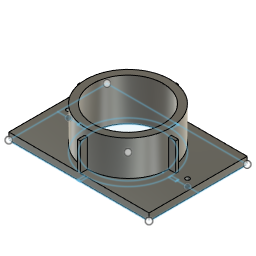
Soporte v1 (Autodesk Fusion 360 design; units mm, degrees)
Autodesk Fusion 360 part; units mm, degrees
sketch "Boceto1" plane through (0, 0, 0) normal (0, 0, 1) x (1, 0, 0)
  circle A0 centre (14.4542, 45.9008) radius 25
  circle A1 centre (14.4542, 45.9008) radius 30
  line L0 (14.4542, 10.9008) -> (15.4542, 10.9008)
  line L1 (15.4542, 10.9008) -> (15.4542, 15.9174)
  line L2 (14.4542, 10.9008) -> (13.4542, 10.9008)
  line L3 (-35.5458, 10.9008) -> (-35.5458, 80.9008)
  line L4 (14.4542, 80.9008) -> (15.4542, 80.9008)
  line L5 (15.4542, 80.9008) -> (15.4542, 75.8841)
  line L6 (15.4542, 80.9008) -> (13.4542, 80.9008)
  line L7 (13.4542, 80.9008) -> (13.4542, 75.8841)
  line L8 (64.4542, 10.9008) -> (64.4542, 80.9008)
  line L9 (14.4542, 10.9008) -> (-35.5458, 10.9008)
  line L10 (14.4542, 10.9008) -> (64.4542, 10.9008)
  line L11 (14.4542, 80.9008) -> (-35.5458, 80.9008)
  line L12 (14.4542, 80.9008) -> (64.4542, 80.9008)
  line L13 (-20.5458, 45.9008) -> (-20.5458, 46.9008)
  line L14 (-20.5458, 46.9008) -> (-15.5291, 46.9008)
  line L15 (-20.5458, 45.9008) -> (-20.5458, 44.9008)
  line L16 (-20.5458, 44.9008) -> (-15.5291, 44.9008)
  line L17 (-20.5458, 45.9008) -> (-35.5458, 45.9008)
  circle A2 centre (-28.0458, 45.9008) radius 1.5
  line L18 (49.4542, 45.9008) -> (49.4542, 46.9008)
  line L19 (49.4542, 46.9008) -> (44.4375, 46.9008)
  line L20 (49.4542, 45.9008) -> (49.4542, 44.9008)
  line L21 (49.4542, 44.9008) -> (44.4375, 44.9008)
  line L22 (49.4542, 45.9008) -> (64.4542, 45.9008)
  circle A3 centre (56.9542, 45.9008) radius 1.5
  line L23 (13.4542, 10.9008) -> (13.4542, 15.9174)
  dimension "d1" = 50
  dimension "d2" = 60
  dimension "d7" = 70
  dimension "d8" = 1
  dimension "d9" = 2
  dimension "d21" = 70
  dimension "d30" = 50
  dimension "d31" = 50
  dimension "d32" = 50
  dimension "d33" = 50
  dimension "d39" = 3
  dimension "d40" = 5.0167
  dimension "d44" = 5.0167
  dimension "d45" = 3
  constraint concentric A0 A1
  constraint coincident A1 L1.end
  constraint perpendicular L0 L1
  constraint coincident A1 L5.end
  constraint perpendicular L4 L5
  constraint coincident A1 L7.end
  constraint parallel L2 L9
  constraint perpendicular L1 L10
  constraint perpendicular L5 L12
  constraint vertical L13
  constraint coincident A1 L14.end
  constraint perpendicular L13 L14
  constraint vertical L15
  constraint coincident A1 L16.end
  constraint perpendicular L15 L16
  constraint midpoint L3 L17.end
  constraint perpendicular L3 L17
  constraint midpoint L17 A2.centre
  constraint coincident A1 L19.end
  constraint perpendicular L18 L19
  constraint coincident A1 L21.end
  constraint perpendicular L18 L21
  constraint midpoint L8 L22.end
  constraint perpendicular L8 L22
  constraint midpoint L22 A3.centre
  constraint coincident A1 L23.end
  constraint perpendicular L9 L23
  measures "d1" diameter of A0
  measures "d2" diameter of A1
  measures "d7" distance of L3.start L3.end
  measures "d8" distance of L4.start L4.end
  measures "d9" distance of L4.end L6.end
  measures "d21" distance of L8.start L8.end
  measures "d30" distance of L0.start L3.start
  measures "d31" distance of L0.start L8.start
  measures "d32" distance of L4.start L3.end
  measures "d33" distance of L4.start L8.end
  measures "d39" diameter of A2
  measures "d40" distance of L15.end L16.end
  measures "d44" distance of L20.end L21.end
  measures "d45" diameter of A3
extrude "Extruir1" add sketch "Boceto1" along normal blind 30 contours A1
extrude "Extruir2" add sketch "Boceto1" along normal blind 25 contours A1 L18 L19 L20 L21 | A1 L4 L5 L6 L7 L11 L12 | A1 L0 L1 L2 L9 L10 L23 | A1 L13 L14 L15 L16
extrude "Extruir3" add sketch "Boceto1" along normal blind 5 contours A1 L5 L8 L12 L18 L19 L22 A3 | A1 L1 L8 L10 L20 L21 L22 A3 | A1 L3 L7 L11 L13 L14 L17 A2 | A1 L3 L9 L15 L16 L17 A2 L23
